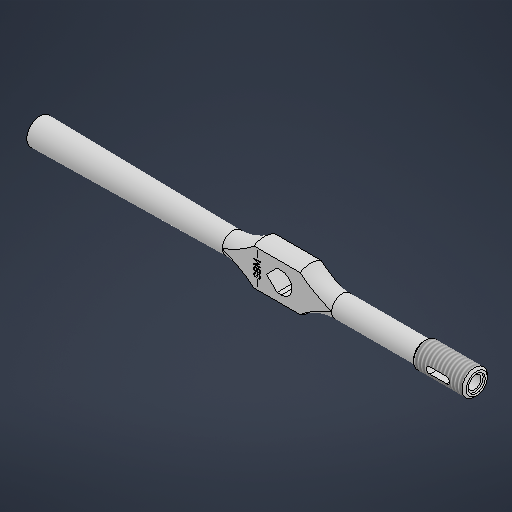
# Autodesk Inventor part: TW1-001
Saved by Autodesk Inventor 2025.3 (Build 293356000, 356)
## iProperties
Created: 2025-05-04
Part Number: TW1-001
Material: Generic
Document SubType Name: Modeling
Designer: fablabadmin
Density: 1 g/cm^3
Appearance: Default
Description: Body
Stock Number: C45E
Author: Benjamin Solar
Title: WEDU
Revision Number: 1
Autodesk Inventor part; units mm, degrees
ref_plane "YZ Plane" through (0, 0, 0) normal (1, 0, 0) x (0, 1, 0)
ref_plane "XZ Plane" through (0, 0, 0) normal (0, 1, 0) x (-1, 0, 0)
ref_plane "XY Plane" through (0, 0, 0) normal (0, 0, 1) x (1, 0, 0)
sketch "Sketch1" plane through (0, 0, 0) normal (0, 0, 1) x (1, 0, 0)
  line L0 (-162.6283, 0) -> (132.1047, 0) projected
  line L1 (0, -12.0245) -> (0, 37.0041) construction
  line L2 (-5.0205, 0) -> (0, 5.0205)
  line L3 (0, -5.0205) -> (-5.0205, 0)
  line L4 (0, 5.0205) -> (2.0795, 5.0205)
  arc A0 (2.0795, -5.0205) -> (2.0795, 5.0205) centre (2.0795, 0) ccw
  line L5 (0, -5.0205) -> (2.0795, -5.0205)
  line L6 (0, 10) -> (-11, 10)
  arc A1 (-26, 5) -> (-11, 10) centre (-26, 30) ccw
  line L7 (-26, 5) -> (-117.8442, 6.2023)
  line L8 (-117.8442, 6.2023) -> (-117.8442, 0)
  line L9 (-26, 5) -> (-117.8442, 5) construction
  line L10 (0, 10) -> (11, 10)
  arc A2 (11, 10) -> (26, 5) centre (26, 30) ccw
  line L11 (26, 5) -> (65, 5)
  line L12 (90, 3) -> (6.1051, 3)
  line L13 (65, 5) -> (66, 6)
  line L14 (89, 6) -> (90, 5)
  line L15 (90, 5) -> (90, 3)
  line L16 (66, 6) -> (89, 6)
  line L17 (77.5, 6) -> (77.5, 3) construction
  line L18 (73.5, 0) -> (81.5, 0) construction
  line L19 (73.5, 1.5) -> (81.5, 1.5)
  line L20 (81.5, -1.5) -> (73.5, -1.5)
  arc A3 (73.5, 1.5) -> (73.5, -1.5) centre (73.5, 0) ccw
  arc A4 (81.5, -1.5) -> (81.5, 1.5) centre (81.5, 0) ccw
  arc A5 (-117.8442, 6.2023) -> (-120, 0) centre (-110, 0) ccw
  line L21 (90, 3) -> (89, 3)
  line L22 (89, 3) -> (89, 4)
  line L23 (89, 4) -> (90, 4)
  line L24 (90, 4) -> (90, 3)
  circle A6 centre (2.0795, 0) radius 5.0205 construction
  point P0 (0, 0)
  point P1 (0, 0)
  point P2 (7.1, 0)
  point P3 (77.5, 0)
  dimension "d0" = 7.1
  dimension "d3" = 2.0795
  dimension "d4" = 0.75
  dimension "d6" = 52
  dimension "d7" = 10
  dimension "d8" = 20
  dimension "d11" = 4.9795
  dimension "d17" = 6
  dimension "d21" = 1
  dimension "d24" = 1
  dimension "d25" = 12
  dimension "d26" = 1
  dimension "d27" = 1
  dimension "d28" = 90
  dimension "d29" = 25
  dimension "d33" = 3
  dimension "d34" = 8
  dimension "d40" = 10
  dimension "d41" = 12.4046
  dimension "d42" = 120
  dimension "d46" = 8
  dimension "d47" = 1
  dimension "d48" = 50
  constraints: 48 end point, 13 point on circle, 6 centre point, 6 tangent, 5 point on line, 4 horizontal, 4 parallel, 4 perpendicular, 3 symmetric about line, 2 coincident, 2 midpoint, 2 vertical, 1 vertical alignment, 16 other
  measures "d0" distance of L2.start L2.end
  measures "d3" distance of L2.end L4.end
  measures "d4" angle of L9 L7
  measures "d6" distance of L11.start L7.start
  measures "d11" distance between parallel lines of L4 L10
  measures "d21" horizontal distance of L13.end L11.end
  measures "d24" horizontal distance of L14.start L14.end
  measures "d26" distance between parallel lines of L16 L11
  measures "d27" distance from line of L14.end L16
  measures "d28" distance between parallel lines of L1 L15
  measures "d29" distance of L14.end L11.end
  measures "d33" distance between parallel lines of L20 L19
  measures "d34" distance of L18.end L18.start
  measures "d40" radius of A5
  measures "d42" distance from line of L1 A5.end
  measures "d47" distance of L22.end L23.end
  measures "d48" diameter of A1
revolve "Revolution1" add sketch "Sketch1" angle 360 about axis through (-10, 0, 0) along (1, 0, 0) contours A5 L8 L0 | L8 L7 A1 L6 L10 A2 L11 L13 L16 L14 L15 L23 L22 L12 A0 L4 L2 L0 | L2 L4 A0 L0
extrude "Extrusion1" cut sketch "Sketch1" along normal through all both and the other way through all contours L2 L4 A0 L0 | L0 A0 L5 L3 | A3 L19 A4 L0 | L0 A4 L20 A3
sketch "Sketch2" plane through (0, 0, 0) normal (0, 1, 0) x (-1, 0, 0)
  line L0 (36.4, 0) -> (-36.4, 0) construction
  line L1 (26, 5) -> (26, -5) construction
  line L2 (-26, 5) -> (-26, -5) construction
  line L3 (26, 10) -> (-26, 10)
  line L4 (-26, 10) -> (-26, 5)
  line L5 (-26, 5) -> (26, 5)
  line L6 (26, 5) -> (26, 10)
  line L7 (11, 10) -> (11, -10) construction
  line L8 (26, -10) -> (-26, -10)
  line L9 (-26, -10) -> (-26, -5)
  line L10 (-26, -5) -> (26, -5)
  line L11 (26, -5) -> (26, -10)
  point P0 (0, 0)
  dimension "d37" = 10
  constraints: 16 end point, 4 point on line, 4 symmetric about line, 2 parallel, 1 horizontal, 1 perpendicular
  measures "d37" distance between parallel lines of L10 L5
extrude "Extrusion2" cut sketch "Sketch2" along normal through all both and the other way through all
thread "Thread1" size "M12x1.75" class "6g" standard "ISO Metric profile" full length
sketch "Sketch4" plane through (-11, -8.6603, 5) normal (0, 0, 1) x (1, 0, 0)
  line L0 (5.9795, 8.6603) -> (11, 3.6398) construction
  line L1 (11, 13.6807) -> (5.9795, 8.6603) construction
  line L2 (13.0795, 13.6807) -> (11, 13.6807) construction
  arc A0 (13.0795, 3.6398) -> (13.0795, 13.6807) centre (13.0795, 8.6603) ccw construction
  line L3 (11, 3.6398) -> (13.0795, 3.6398) construction
  line L4 (22, 0) -> (0, 0) construction
  line L5 (0, 17.3205) -> (22, 17.3205) construction
  line L6 (-151, 8.6603) -> (143, 8.6603) construction
  line L7 (1.5, 8.6603) -> (1.5, 17.3205) construction
  line L8 (1.5, 13.0366) -> (1.5, 16.2606)
  line L9 (1.5, 4.2839) -> (1.5, 1.0599)
  point P0 (11, 8.6603)
  dimension "d45" = 9.5
  constraints: 6 end point, 4 point on line, 2 symmetric about line, 1 perpendicular, 5 other
  measures "d45" distance of point (11, 8.66) L7.start
mark "Mark2"
equation "\"d21\" = d26"
equation "\"d24\" = d26"
equation "\"d27\" = d24"
body "Solid1"
